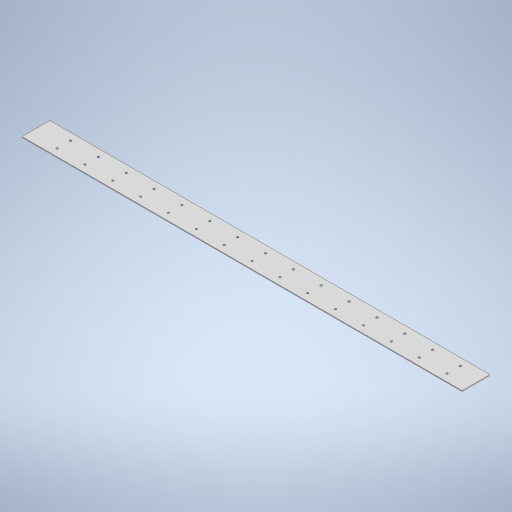
# Autodesk Inventor part: Sketch-3-44
Saved by Autodesk Inventor 2023 (Build 270158000, 158)
## iProperties
Created: 2023-02-21
Part Number: Sketch-3-44
Material: Generic
Document SubType Name: Sheet Metal
Designer: emila
Density: 1 g/cm^3
Appearance: Default
Sheet Metal Rule: Default_mm
Author: emila
Autodesk Inventor part; units mm, degrees
ref_plane "YZ Plane" through (0, 0, 0) normal (1, 0, 0) x (0, 1, 0)
ref_plane "XZ Plane" through (0, 0, 0) normal (0, 1, 0) x (-1, 0, 0)
ref_plane "XY Plane" through (0, 0, 0) normal (0, 0, 1) x (1, 0, 0)
sketch "Sketch2" plane through (0, 0, 0) normal (0, 1, 0) x (-1, 0, 0)
  line L0 (51.7371, 79.6504) -> (-734.2629, 79.6504)
  line L1 (-736.2629, 77.6504) -> (-736.2629, 31.6504)
  line L2 (-734.2629, 29.6504) -> (51.7371, 29.6504)
  line L3 (53.7371, 31.6504) -> (53.7371, 77.6504)
  arc A0 (51.7371, 29.6504) -> (53.7371, 31.6504) centre (51.7371, 31.6504) ccw
  arc A1 (53.7371, 77.6504) -> (51.7371, 79.6504) centre (51.7371, 77.6504) ccw
  arc A2 (-734.2629, 79.6504) -> (-736.2629, 77.6504) centre (-734.2629, 77.6504) ccw
  arc A3 (-736.2629, 31.6504) -> (-734.2629, 29.6504) centre (-734.2629, 31.6504) ccw
  point P0 (0, 0)
  point P1 (53.7371, 79.6504)
  point P2 (-736.2629, 29.6504)
  point P3 (-736.2629, 79.6504)
  point P4 (53.7371, 29.6504)
  dimension "d11" = 50
  dimension "d33" = 790
  dimension "d34" = 2
  measures "d11" distance of point (53.737, 29.65) point (53.737, 79.65)
  measures "d33" distance of point (-736.263, 29.65) point (53.737, 29.65)
  measures "d34" radius of A0
extrude "Plate1" add sketch "Sketch2" along normal blind 1.5
sketch "Sketch5" plane through (0, 1.5, 0) normal (0, 1, 0) x (1, 0, 0)
  line L0 (-53.7371, -77.6504) -> (-53.7371, -31.6504) projected
  line L1 (-53.7371, -54.6504) -> (736.2629, -54.6504) construction
  line L2 (736.2629, -31.6504) -> (736.2629, -77.6504) projected
  circle A0 centre (-3.7371, -42.6504) radius 1.7
  circle A1 centre (-3.7371, -66.6504) radius 1.7
  line L3 (-3.7371, -54.6504) -> (786.2629, -54.6504) construction
  circle A2 centre (46.2629, -42.6504) radius 1.7
  circle A3 centre (46.2629, -66.6504) radius 1.7
  line L4 (46.2629, -54.6504) -> (836.2629, -54.6504) construction
  circle A4 centre (96.2629, -42.6504) radius 1.7
  circle A5 centre (96.2629, -66.6504) radius 1.7
  line L5 (96.2629, -54.6504) -> (886.2629, -54.6504) construction
  circle A6 centre (146.2629, -42.6504) radius 1.7
  circle A7 centre (146.2629, -66.6504) radius 1.7
  line L6 (146.2629, -54.6504) -> (936.2629, -54.6504) construction
  circle A8 centre (196.2629, -42.6504) radius 1.7
  circle A9 centre (196.2629, -66.6504) radius 1.7
  line L7 (196.2629, -54.6504) -> (986.2629, -54.6504) construction
  circle A10 centre (246.2629, -42.6504) radius 1.7
  circle A11 centre (246.2629, -66.6504) radius 1.7
  line L8 (246.2629, -54.6504) -> (1036.2629, -54.6504) construction
  circle A12 centre (296.2629, -42.6504) radius 1.7
  circle A13 centre (296.2629, -66.6504) radius 1.7
  line L9 (296.2629, -54.6504) -> (1086.2629, -54.6504) construction
  circle A14 centre (346.2629, -42.6504) radius 1.7
  circle A15 centre (346.2629, -66.6504) radius 1.7
  line L10 (346.2629, -54.6504) -> (1136.2629, -54.6504) construction
  circle A16 centre (396.2629, -42.6504) radius 1.7
  circle A17 centre (396.2629, -66.6504) radius 1.7
  line L11 (396.2629, -54.6504) -> (1186.2629, -54.6504) construction
  circle A18 centre (446.2629, -42.6504) radius 1.7
  circle A19 centre (446.2629, -66.6504) radius 1.7
  line L12 (446.2629, -54.6504) -> (1236.2629, -54.6504) construction
  circle A20 centre (496.2629, -42.6504) radius 1.7
  circle A21 centre (496.2629, -66.6504) radius 1.7
  line L13 (496.2629, -54.6504) -> (1286.2629, -54.6504) construction
  circle A22 centre (546.2629, -42.6504) radius 1.7
  circle A23 centre (546.2629, -66.6504) radius 1.7
  line L14 (546.2629, -54.6504) -> (1336.2629, -54.6504) construction
  circle A24 centre (596.2629, -42.6504) radius 1.7
  circle A25 centre (596.2629, -66.6504) radius 1.7
  line L15 (596.2629, -54.6504) -> (1386.2629, -54.6504) construction
  circle A26 centre (646.2629, -42.6504) radius 1.7
  circle A27 centre (646.2629, -66.6504) radius 1.7
  line L16 (646.2629, -54.6504) -> (1436.2629, -54.6504) construction
  circle A28 centre (696.2629, -42.6504) radius 1.7
  circle A29 centre (696.2629, -66.6504) radius 1.7
  point P0 (0, 0)
  dimension "d35" = 3.4
  dimension "d36" = 12
  dimension "d37" = 50
  dimension "d40" = 50
  constraints: 30 centre point, 30 end point, 2 midpoint, 1 collinear, 1 horizontal, 1 symmetric about line, 98 other
  measures "d35" diameter of A0
  measures "d36" distance from line of L1 A0.centre
  measures "d37" distance from line of L0 A0.centre
  measures "d40" distance of L1.start L3.start
hole "Hole1" at (-3.7371, 1.5, 42.6504) at (-3.7371, 1.5, 66.6504) at (46.2629, 1.5, 42.6504) at (46.2629, 1.5, 66.6504) at (96.2629, 1.5, 42.6504) at (96.2629, 1.5, 66.6504) at (146.2629, 1.5, 42.6504) at (146.2629, 1.5, 66.6504) at (196.2629, 1.5, 42.6504) at (196.2629, 1.5, 66.6504) at (246.2629, 1.5, 42.6504) at (246.2629, 1.5, 66.6504) at (296.2629, 1.5, 42.6504) at (296.2629, 1.5, 66.6504) at (346.2629, 1.5, 42.6504) at (346.2629, 1.5, 66.6504) at (396.2629, 1.5, 66.6504) at (396.2629, 1.5, 42.6504) at (446.2629, 1.5, 42.6504) at (446.2629, 1.5, 66.6504) at (496.2629, 1.5, 42.6504) at (496.2629, 1.5, 66.6504) at (546.2629, 1.5, 66.6504) at (546.2629, 1.5, 42.6504) at (596.2629, 1.5, 42.6504) at (596.2629, 1.5, 66.6504) at (646.2629, 1.5, 66.6504) at (646.2629, 1.5, 42.6504) at (696.2629, 1.5, 42.6504) at (696.2629, 1.5, 66.6504) direction (0, -1, 0) diameter 3.4 end through all
equation "\"d50\" = Thickness"
equation "\"d12\" = Thickness"
equation "\"BendRadius\" = Thickness"
equation "\"BendReliefWidth\" = Thickness"
equation "\"BendReliefDepth\" = 0.5 * Thickness"
equation "\"CornerReliefSize\" = 4 * Thickness"
equation "\"MinimumRemnant\" = 2 * Thickness"
equation "\"TransitionRadius\" = BendRadius"
equation "\"JacobiRadiusSize\" = BendRadius"
equation "\"GapSize\" = Thickness"
equation "\"Thickness\" = 1.5"
body "Solid1"
